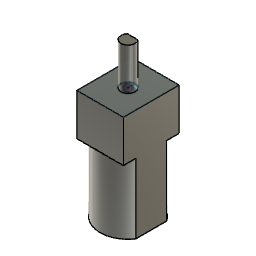
N20 Motor v3 (Autodesk Fusion 360 design; units mm, degrees)
Autodesk Fusion 360 part; units mm, degrees
note: some values were not read from the file. Set by a fixed rule: which sketch regions a step uses.
sketch "Sketch1" plane through (0, 0, 0) normal (0, 0, 1) x (1, 0, 0)
  circle A0 centre (0, 0) radius 6
  line L0 (5, -7) -> (-5, -7)
  line L1 (-5, -7) -> (-5, 7)
  line L2 (-5, 7) -> (5, 7)
  line L3 (5, 7) -> (5, -7)
  line L4 (5, -7) -> (-5, 7) construction
  line L5 (-5, -7) -> (5, 7) construction
  dimension "d1" = 12
  constraint coincident A0.centre origin
  constraint horizontal L0
  constraint perpendicular L0 L1
  constraint parallel L0 L2
  constraint parallel L1 L3
  constraint coincident L4 A0.centre
  constraint coincident L5 A0.centre
  measures "d1" diameter of A0
extrude "Extrude1" add sketch "Sketch1" along normal blind 15 contours A0 L1 L3
sketch "Sketch2" plane through (0, 0, 0) normal (0, 0, 1) x (1, 0, 0)
  line L0 (5, -6) -> (-5, -6)
  line L1 (-5, -6) -> (-5, 6)
  line L2 (-5, 6) -> (5, 6)
  line L3 (5, 6) -> (5, -6)
  line L4 (5, -6) -> (-5, 6) construction
  line L5 (-5, -6) -> (5, 6) construction
  constraint horizontal L0
  constraint perpendicular L0 L1
  constraint parallel L0 L2
  constraint parallel L1 L3
  constraint coincident L4 origin
  constraint coincident L5 origin
sketch "Sketch3" plane through (0, 0, 0) normal (0, 0, 1) x (1, 0, 0)
sketch "Sketch4" plane through (0, 0, 0) normal (0, 0, 1) x (1, 0, 0)
sketch "Sketch5" plane through (0, 0, 15) normal (0, 0, 1) x (-1, 0, 0)
  arc A0 (5, 3.3166) -> (-5, 3.3166) centre (0, 0) ccw
  line L0 (-5, 3.3166) -> (-5, -3.3166)
  arc A1 (-5, -3.3166) -> (5, -3.3166) centre (0, 0) ccw
  line L1 (5, -3.3166) -> (5, 3.3166)
  line L2 (-5, 6) -> (5, 6)
  line L3 (5, 6) -> (5, -6)
  line L4 (5, -6) -> (-5, -6)
  line L5 (-5, -6) -> (-5, 6)
  line L6 (-5, 6) -> (5, -6) construction
  line L7 (5, 6) -> (-5, -6) construction
  constraint horizontal L2
  constraint perpendicular L2 L3
  constraint parallel L2 L4
  constraint parallel L3 L5
  constraint coincident L6 A0.centre
  constraint coincident L7 A0.centre
  constraint coincident A0.centre A1.centre
extrude "Extrude2" add sketch "Sketch5" along normal blind 9
sketch "Sketch6" plane through (0, 0, 24) normal (0, 0, 1) x (-1, 0, 0)
  line L0 (-5, -6) -> (5, -6)
  line L1 (5, -6) -> (5, 6)
  line L2 (5, 6) -> (-5, 6)
  line L3 (-5, 6) -> (-5, -6)
  circle A0 centre (0, 0) radius 1.5
  line L4 (0, 0) -> (0, -1)
  line L5 (0, -1) -> (-1.118, -1)
  line L6 (0, -1) -> (1.118, -1)
  line L7 (1.118, -1) -> (-1.118, -1)
  dimension "d6" = 3
  constraint coincident A0.centre L4.start
  constraint vertical L4
  constraint coincident A0 L5.end
  constraint perpendicular L4 L5
  constraint coincident A0 L6.end
  constraint perpendicular L4 L6
  measures "d6" diameter of A0
extrude "Extrude3" add sketch "Sketch6" along normal blind 9 contours A0 L5 L6 L7 picked at (0.0074, 0.6639)
extrude "Extrude5" add sketch "Sketch6" along normal blind 2 contours A0 L5 L6 L7 picked at (0.0699, -1.3284)
extrude "Extrude4" [suppressed]
